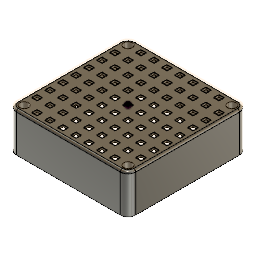
box (Autodesk Fusion 360 design; units mm, degrees)
Autodesk Fusion 360 part; units mm, degrees
sketch "Sketch1" plane through (0, 0, 0) normal (0, 0, 1) x (1, 0, 0) in component "Bottom"
  line L0 (50, 55) -> (-50, 55)
  line L1 (-55, 50) -> (-55, -50)
  line L2 (-50, -55) -> (50, -55)
  line L3 (55, -50) -> (55, 50)
  line L4 (55, 55) -> (-55, -55) construction
  line L5 (-55, 55) -> (55, -55) construction
  arc A0 (-50, 55) -> (-55, 50) centre (-50, 50) ccw
  arc A1 (55, 50) -> (50, 55) centre (50, 50) ccw
  arc A2 (50, -55) -> (55, -50) centre (50, -50) ccw
  arc A3 (-55, -50) -> (-50, -55) centre (-50, -50) ccw
  circle A4 centre (-50, 50) radius 2.25
  circle A5 centre (-50, 50) radius 5.85
  circle A6 centre (50, 50) radius 2.25
  circle A7 centre (50, 50) radius 5.85
  circle A8 centre (-50, -50) radius 2.25
  circle A9 centre (-50, -50) radius 5.85
  circle A10 centre (50, -50) radius 2.25
  circle A11 centre (50, -50) radius 5.85
  dimension "d1" = 110
  dimension "d2" = 110
  dimension "d3" = 5
  dimension "d33" = 4.5
  dimension "d34" = 3.6
  dimension "d37" = 100
  dimension "d38" = -100
  dimension "d39" = 5
  constraint perpendicular L0 L1
  constraint parallel L0 L2
  constraint parallel L1 L3
  constraint horizontal L0
  constraint coincident L4 origin
  constraint coincident L5 origin
  constraint coincident L5.start L1
  constraint coincident L5.start L0
  constraint tangent L1 A0
  constraint tangent L0 A0
  constraint coincident L4.start L0
  constraint coincident L4.start L3
  constraint tangent L0 A1
  constraint tangent L3 A1
  constraint equal A0 A1
  constraint coincident L5.end L3
  constraint coincident L5.end L2
  constraint tangent L3 A2
  constraint tangent L2 A2
  constraint equal A0 A2
  constraint coincident L4.end L2
  constraint coincident L4.end L1
  constraint tangent L2 A3
  constraint tangent L1 A3
  constraint equal A0 A3
  constraint coincident L5 A0.centre
  measures "d1" distance of L5.start L4.end
  measures "d2" distance of L4.end L5.end
  measures "d3" radius of A0
  measures "d33" diameter of A4
  measures "d39" distance of L1 A0.centre
extrude "Extrude1" add sketch "Sketch1" along normal blind 2 contours L0 L3 A1 A7 | L0 L1 L2 L3 A5 A7 A9 A11 | L0 L1 A0 A5 | L2 L3 A2 A11 | L1 L2 A3 A9 picked at (54.0091, 48.6623) picked at (-54.0091, 48.6623) picked at (54.0091, -48.6623) picked at (-54.0091, -48.6623) makes body 1 in component "Bottom"
sketch "Sketch2" plane through (0, 0, 2) normal (0, 0, 1) x (-1, 0, 0) in component "Bottom"
  arc A0 (55, 50) -> (50, 55) centre (50, 50) ccw
  line L0 (50, 55) -> (-50, 55)
  arc A1 (-50, 55) -> (-55, 50) centre (-50, 50) ccw
  line L1 (-55, 50) -> (-55, -50)
  arc A2 (-55, -50) -> (-50, -55) centre (-50, -50) ccw
  line L2 (-50, -55) -> (50, -55)
  arc A3 (50, -55) -> (55, -50) centre (50, -50) ccw
  line L3 (55, -50) -> (55, 50)
  line L4 (44, 50) -> (-44, 50)
  line L5 (-44, 50) -> (-44, 10.8)
  line L6 (-44, 10.8) -> (44, 10.8)
  line L7 (44, 10.8) -> (44, 50)
  line L8 (44, 50) -> (-44, 10.8) construction
  line L9 (-44, 50) -> (44, 10.8) construction
  line L10 (0, -55) -> (0, 55) construction
  line L11 (50, 55) -> (-50, 55)
  line L12 (-37.8, 44.5) -> (37.8, 44.5) construction
  line L13 (37.8, 44.5) -> (37.8, 16.3) construction
  line L14 (37.8, 16.3) -> (-37.8, 16.3) construction
  line L15 (-37.8, 16.3) -> (-37.8, 44.5) construction
  line L16 (-37.8, 44.5) -> (37.8, 16.3) construction
  line L17 (37.8, 44.5) -> (-37.8, 16.3) construction
  circle A4 centre (37.8, 16.3) radius 1.5
  circle A5 centre (-37.8, 44.5) radius 1.5
  line L18 (-41.5, 7) -> (41.5, 7)
  line L19 (41.5, 7) -> (41.5, -50)
  line L20 (41.5, -50) -> (-41.5, -50)
  line L21 (-41.5, -50) -> (-41.5, 7)
  line L22 (-41.5, 7) -> (41.5, -50) construction
  line L23 (41.5, 7) -> (-41.5, -50) construction
  line L24 (-50, -55) -> (50, -55)
  line L25 (45, 10.5) -> (45, -53.5) construction
  line L26 (45, -53.5) -> (-45, -53.5) construction
  line L27 (-45, -53.5) -> (-45, 10.5) construction
  line L28 (-45, 10.5) -> (45, 10.5) construction
  circle A6 centre (-45, -9) radius 1.5
  circle A7 centre (45, -34) radius 1.5
  line L29 (-45, -13.5) -> (-41.5, -13.5)
  line L30 (-45, -4.5) -> (-41.5, -4.5)
  arc A8 (-45, -4.5) -> (-45, -13.5) centre (-45, -9) ccw
  line L31 (45, -38.5) -> (41.5, -38.5)
  line L32 (45, -29.5) -> (41.5, -29.5)
  arc A9 (45, -38.5) -> (45, -29.5) centre (45, -34) ccw
  circle A10 centre (50, -50) radius 2.25
  circle A11 centre (-50, -50) radius 2.25
  circle A12 centre (50, 50) radius 2.25
  circle A13 centre (-50, 50) radius 2.25
  point P0 (0, 30.4)
  point P1 (0, 30.4)
  point P2 (0, -21.5)
  dimension "d6" = 88
  dimension "d7" = 39.2
  dimension "d9" = 5
  dimension "d10" = 28.2
  dimension "d11" = 75.6
  dimension "d12" = 3
  dimension "d13" = 3
  dimension "d19" = 57
  dimension "d20" = 83
  dimension "d21" = 5
  dimension "d22" = -3.5
  dimension "d23" = 3
  dimension "d24" = 16
  dimension "d25" = 3
  dimension "d26" = 16
  constraint perpendicular L4 L5
  constraint parallel L4 L6
  constraint parallel L5 L7
  constraint coincident L8 P1
  constraint coincident L9 P1
  constraint midpoint L2 L10.start
  constraint midpoint L0 L10.end
  constraint coincident P1 L10
  constraint vertical L5
  constraint perpendicular L12 L13
  constraint parallel L12 L14
  constraint parallel L13 L15
  constraint horizontal L12
  constraint coincident L16 P1
  constraint coincident L17 P1
  constraint coincident P1 P0
  constraint coincident L13.end L14.start
  constraint coincident L12.start L15.end
  constraint perpendicular L18 L19
  constraint parallel L18 L20
  constraint parallel L19 L21
  constraint horizontal L18
  constraint coincident L22 P2
  constraint coincident L23 P2
  constraint coincident L10 P2
  constraint coincident L27 A6.centre
  constraint coincident L25 A7.centre
  constraint coincident L27 L29.start
  constraint coincident L21 L29.end
  constraint tangent L29 A8
  constraint perpendicular L21 L29
  constraint coincident L27 L30.start
  constraint coincident L21 L30.end
  constraint tangent L30 A8
  constraint perpendicular L21 L30
  constraint concentric A6 A8
  constraint coincident L25 L31.start
  constraint coincident L19 L31.end
  constraint tangent L31 A9
  constraint perpendicular L19 L31
  constraint coincident L25 L32.start
  constraint coincident L19 L32.end
  constraint tangent L32 A9
  constraint perpendicular L19 L32
  constraint concentric A7 A9
  measures "d6" distance of L5.end L6.end
  measures "d7" distance of L4.end L5.end
  measures "d9" distance of L4 L11
  measures "d10" distance of L12.end L13.end
  measures "d11" distance of L13 L15
  measures "d12" diameter of A4
  measures "d13" diameter of A5
  measures "d19" distance of L18.end L19.end
  measures "d20" distance of L19.end L20.end
  measures "d21" distance of L20 L24
  measures "d23" diameter of A6
  measures "d24" vertical distance of L18.start A6.centre
  measures "d25" diameter of A7
  measures "d26" distance of L20 A7.centre
extrude "Extrude2" add sketch "Sketch2" along normal blind 1 contours L18 L19 L20 L21 | L21 L29 L30 A8 | L19 L31 L32 A9 bodies 1 in component "Bottom"
extrude "Extrude4" add sketch "Sketch2" along normal blind 3 contours L4 L5 L6 L7 bodies 1 in component "Bottom"
fillet "Fillet2" radius 4 4 edges at (44, -10.8, 3.5) (-44, -10.8, 3.5) (-44, -50, 3.5) (44, -50, 3.5) on bodies 1 in component "Bottom"
extrude "Extrude5" cut sketch "Sketch2" against normal through all contours A4 | A5 | A6 | A7 bodies 1 in component "Bottom"
ref_plane "WorkPlane1" through (0, 0, 36) normal (0, 0, 1) x (-1, 0, 0) in component "Cover"
sketch "Sketch1 (2)" plane through (0, 0, 36) normal (0, 0, 1) x (1, 0, 0) in component "Cover"
  circle A0 centre (37.8, -44.5) radius 1.5
  circle A1 centre (45, 9) radius 1.5
  circle A2 centre (-37.8, -16.3) radius 1.5
  circle A3 centre (-45, 34) radius 1.5
  circle A4 centre (-50, -50) radius 2.25
  circle A5 centre (-50, 50) radius 2.25
  circle A6 centre (50, -50) radius 2.25
  circle A7 centre (50, 50) radius 2.25
  arc A8 (-55, -50) -> (-50, -55) centre (-50, -50) ccw
  line L0 (-55, -50) -> (-55, 50)
  arc A9 (-50, 55) -> (-55, 50) centre (-50, 50) ccw
  line L1 (-50, 55) -> (50, 55)
  arc A10 (55, 50) -> (50, 55) centre (50, 50) ccw
  line L2 (55, 50) -> (55, -50)
  arc A11 (50, -55) -> (55, -50) centre (50, -50) ccw
  line L3 (50, -55) -> (-50, -55)
  arc A12 (-55.4, -50) -> (-50, -55.4) centre (-50, -50) ccw
  line L4 (50, -55.4) -> (-50, -55.4)
  arc A13 (50, -55.4) -> (55.4, -50) centre (50, -50) ccw
  line L5 (55.4, 50) -> (55.4, -50)
  arc A14 (55.4, 50) -> (50, 55.4) centre (50, 50) ccw
  line L6 (-50, 55.4) -> (50, 55.4)
  arc A15 (-50, 55.4) -> (-55.4, 50) centre (-50, 50) ccw
  line L7 (-55.4, -50) -> (-55.4, 50)
  arc A16 (-57.4, -50) -> (-50, -57.4) centre (-50, -50) ccw
  line L8 (50, -57.4) -> (-50, -57.4)
  arc A17 (50, -57.4) -> (57.4, -50) centre (50, -50) ccw
  line L9 (57.4, 50) -> (57.4, -50)
  arc A18 (57.4, 50) -> (50, 57.4) centre (50, 50) ccw
  line L10 (-50, 57.4) -> (50, 57.4)
  arc A19 (-50, 57.4) -> (-57.4, 50) centre (-50, 50) ccw
  line L11 (-57.4, -50) -> (-57.4, 50)
  dimension "d41" = -0.4
  dimension "d42" = -2.4
extrude "Extrude1'" add sketch "Sketch1 (2)" along normal blind 2 separate body contours A0 | A1 | A2 | A3 | A8 L0 A9 L1 A10 L2 A11 L3 | A12 L4 A13 L5 A14 L6 A15 L7 | A16 L8 A17 L9 A18 L10 A19 L11 makes body 2 in component "Cover"
sketch "Sketch2 (2)" plane through (0, 0, 36) normal (0, 0, 1) x (1, 0, 0) in component "Cover"
  circle A0 centre (-50, -50) radius 5.85
  circle A1 centre (50, -50) radius 5.85
  circle A2 centre (50, 50) radius 5.85
  circle A3 centre (-50, 50) radius 5.85
  circle A4 centre (50, -50) radius 2.25 construction
  circle A5 centre (-50, -50) radius 2.25 construction
  circle A6 centre (-50, 50) radius 2.25 construction
  circle A7 centre (50, 50) radius 2.25 construction
  line L0 (-57.4, 50) -> (-57.4, -50)
  line L1 (-57.4, -44.15) -> (-50, -44.15)
  line L2 (50, -57.4) -> (-50, -57.4)
  line L3 (-44.15, -50) -> (-44.15, -57.4)
  line L4 (44.15, -50) -> (44.15, -57.4)
  line L5 (57.4, -50) -> (57.4, 50)
  line L6 (50, -44.15) -> (57.4, -44.15)
  line L7 (50, 44.15) -> (57.4, 44.15)
  line L8 (-50, 57.4) -> (50, 57.4)
  line L9 (44.15, 50) -> (44.15, 57.4)
  line L10 (-50, 44.15) -> (-57.4, 44.15)
  line L11 (-44.15, 50) -> (-44.15, 57.4)
  circle A8 centre (-50, -50) radius 2.25
  circle A9 centre (-50, 50) radius 2.25
  circle A10 centre (50, 50) radius 2.25
  circle A11 centre (50, -50) radius 2.25
  arc A12 (50, -57.4) -> (57.4, -50) centre (50, -50) ccw
  line L12 (50, -57.4) -> (-50, -57.4)
  arc A13 (-57.4, -50) -> (-50, -57.4) centre (-50, -50) ccw
  line L13 (-57.4, -50) -> (-57.4, 50)
  arc A14 (-50, 57.4) -> (-57.4, 50) centre (-50, 50) ccw
  line L14 (-50, 57.4) -> (50, 57.4)
  arc A15 (57.4, 50) -> (50, 57.4) centre (50, 50) ccw
  line L15 (57.4, 50) -> (57.4, -50)
  constraint coincident L0 L1.start
  constraint coincident A0 L1.end
  constraint tangent A0 L1
  constraint perpendicular L0 L1
  constraint coincident A0 L3.start
  constraint coincident L2 L3.end
  constraint tangent A0 L3
  constraint perpendicular L2 L3
  constraint coincident A1 L4.start
  constraint coincident L2 L4.end
  constraint coincident A1 L6.start
  constraint coincident L5 L6.end
  constraint tangent A1 L6
  constraint perpendicular L5 L6
  constraint coincident A2 L7.start
  constraint coincident L5 L7.end
  constraint coincident A2 L9.start
  constraint coincident L8 L9.end
  constraint tangent A2 L9
  constraint perpendicular L8 L9
  constraint coincident A3 L10.start
  constraint coincident L0 L10.end
  constraint coincident A3 L11.start
  constraint coincident L8 L11.end
  constraint tangent A3 L10
  constraint tangent A3 L11
  constraint tangent A2 L7
  constraint tangent A1 L4
  constraint perpendicular L8 L11
  constraint perpendicular L0 L10
  constraint perpendicular L5 L7
  constraint perpendicular L2 L4
extrude "Extrude3" add sketch "Sketch2 (2)" against normal blind 34 contours A0 | A0 L0 L1 L2 L3 L12 A13 L13 | A1 L2 L4 L5 L6 A12 L12 L15 | A3 L0 L8 L10 L11 L13 A14 L14 | A1 | A3 | A2 L5 L7 L8 L9 L14 A15 L15 | A2 bodies 2 in component "Cover"
extrude "Extrude2'" add sketch "Sketch1 (2)" against normal up to surface (36 mm away) contours A16 L8 A17 L9 A18 L10 A19 L11 bodies 2 in component "Cover"
sketch "Sketch3" plane through (0, 0, 38) normal (0, 0, 1) x (-1, 0, 0) in component "Cover"
  circle A0 centre (-50, -50) radius 2.25
  circle A1 centre (-50, 50) radius 2.25
  circle A2 centre (50, -50) radius 2.25
  circle A3 centre (50, 50) radius 2.25
  arc A4 (-50, 57.4) -> (-57.4, 50) centre (-50, 50) ccw
  line L0 (-57.4, 50) -> (-57.4, -50)
  arc A5 (-57.4, -50) -> (-50, -57.4) centre (-50, -50) ccw
  line L1 (-50, -57.4) -> (50, -57.4)
  arc A6 (50, -57.4) -> (57.4, -50) centre (50, -50) ccw
  line L2 (57.4, -50) -> (57.4, 50)
  arc A7 (57.4, 50) -> (50, 57.4) centre (50, 50) ccw
  line L3 (50, 57.4) -> (-50, 57.4)
  circle A8 centre (50, -50) radius 4.1
  circle A9 centre (-50, -50) radius 4.1
  circle A10 centre (50, 50) radius 4.1
  circle A11 centre (-50, 50) radius 4.1
  dimension "d49" = 8.2
  dimension "d50" = 8.2
  dimension "d51" = 8.2
  dimension "d52" = 8.2
  constraint concentric A2 A8
  constraint concentric A0 A9
  constraint concentric A3 A10
  constraint concentric A1 A11
  measures "d49" diameter of A8
  measures "d50" diameter of A9
  measures "d51" diameter of A10
  measures "d52" diameter of A11
extrude "Extrude4'" cut sketch "Sketch3" against normal blind 30 contours A8 | A9 | A10 | A11 bodies 2 in component "Cover"
chamfer "Chamfer1" distance 1.8 angle 45 4 edges at (-52.0977, -50.8136, 8) (-52.0977, 49.1864, 8) (47.9023, 49.1864, 8) (47.9023, -50.8136, 8) on bodies 2 in component "Cover"
sketch "Sketch4" plane through (0, 0, 38) normal (0, 0, 1) x (-1, 0, 0) in component "Cover"
  circle A0 centre (50, -50) radius 4.1
  circle A1 centre (-50, -50) radius 4.1
  circle A2 centre (50, 50) radius 4.1
  circle A3 centre (-50, 50) radius 4.1
  arc A4 (-50, 57.4) -> (-57.4, 50) centre (-50, 50) ccw
  line L0 (-57.4, 50) -> (-57.4, -50)
  arc A5 (-57.4, -50) -> (-50, -57.4) centre (-50, -50) ccw
  line L1 (-50, -57.4) -> (50, -57.4)
  arc A6 (50, -57.4) -> (57.4, -50) centre (50, -50) ccw
  line L2 (57.4, -50) -> (57.4, 50)
  arc A7 (57.4, 50) -> (50, 57.4) centre (50, 50) ccw
  line L3 (50, 57.4) -> (-50, 57.4)
  line L4 (-2.5, -2.5) -> (2.5, -2.5)
  line L5 (2.5, -2.5) -> (2.5, 2.5)
  line L6 (2.5, 2.5) -> (-2.5, 2.5)
  line L7 (-2.5, 2.5) -> (-2.5, -2.5)
  line L8 (-2.5, -2.5) -> (2.5, 2.5) construction
  line L9 (2.5, -2.5) -> (-2.5, 2.5) construction
  line L10 (-35, -52.5) -> (-35, -47.5)
  line L11 (-40, -52.5) -> (-35, -52.5)
  line L12 (-40, -47.5) -> (-40, -52.5)
  line L13 (-35, -47.5) -> (-40, -47.5)
  line L14 (-22.5, -52.5) -> (-22.5, -47.5)
  line L15 (-27.5, -52.5) -> (-22.5, -52.5)
  line L16 (-27.5, -47.5) -> (-27.5, -52.5)
  line L17 (-22.5, -47.5) -> (-27.5, -47.5)
  line L18 (-10, -52.5) -> (-10, -47.5)
  line L19 (-15, -52.5) -> (-10, -52.5)
  line L20 (-15, -47.5) -> (-15, -52.5)
  line L21 (-10, -47.5) -> (-15, -47.5)
  line L22 (2.5, -52.5) -> (2.5, -47.5)
  line L23 (-2.5, -52.5) -> (2.5, -52.5)
  line L24 (-2.5, -47.5) -> (-2.5, -52.5)
  line L25 (2.5, -47.5) -> (-2.5, -47.5)
  line L26 (15, -52.5) -> (15, -47.5)
  line L27 (10, -52.5) -> (15, -52.5)
  line L28 (10, -47.5) -> (10, -52.5)
  line L29 (15, -47.5) -> (10, -47.5)
  line L30 (27.5, -52.5) -> (27.5, -47.5)
  line L31 (22.5, -52.5) -> (27.5, -52.5)
  line L32 (22.5, -47.5) -> (22.5, -52.5)
  line L33 (27.5, -47.5) -> (22.5, -47.5)
  line L34 (40, -52.5) -> (40, -47.5)
  line L35 (35, -52.5) -> (40, -52.5)
  line L36 (35, -47.5) -> (35, -52.5)
  line L37 (40, -47.5) -> (35, -47.5)
  line L38 (-47.5, -40) -> (-47.5, -35)
  line L39 (-52.5, -40) -> (-47.5, -40)
  line L40 (-52.5, -35) -> (-52.5, -40)
  line L41 (-47.5, -35) -> (-52.5, -35)
  line L42 (-35, -40) -> (-35, -35)
  line L43 (-40, -40) -> (-35, -40)
  line L44 (-40, -35) -> (-40, -40)
  line L45 (-35, -35) -> (-40, -35)
  line L46 (-22.5, -40) -> (-22.5, -35)
  line L47 (-27.5, -40) -> (-22.5, -40)
  line L48 (-27.5, -35) -> (-27.5, -40)
  line L49 (-22.5, -35) -> (-27.5, -35)
  line L50 (-10, -40) -> (-10, -35)
  line L51 (-15, -40) -> (-10, -40)
  line L52 (-15, -35) -> (-15, -40)
  line L53 (-10, -35) -> (-15, -35)
  line L54 (2.5, -40) -> (2.5, -35)
  line L55 (-2.5, -40) -> (2.5, -40)
  line L56 (-2.5, -35) -> (-2.5, -40)
  line L57 (2.5, -35) -> (-2.5, -35)
  line L58 (15, -40) -> (15, -35)
  line L59 (10, -40) -> (15, -40)
  line L60 (10, -35) -> (10, -40)
  line L61 (15, -35) -> (10, -35)
  line L62 (27.5, -40) -> (27.5, -35)
  line L63 (22.5, -40) -> (27.5, -40)
  line L64 (22.5, -35) -> (22.5, -40)
  line L65 (27.5, -35) -> (22.5, -35)
  line L66 (40, -40) -> (40, -35)
  line L67 (35, -40) -> (40, -40)
  line L68 (35, -35) -> (35, -40)
  line L69 (40, -35) -> (35, -35)
  line L70 (52.5, -40) -> (52.5, -35)
  line L71 (47.5, -40) -> (52.5, -40)
  line L72 (47.5, -35) -> (47.5, -40)
  line L73 (52.5, -35) -> (47.5, -35)
  line L74 (-47.5, -27.5) -> (-47.5, -22.5)
  line L75 (-52.5, -27.5) -> (-47.5, -27.5)
  line L76 (-52.5, -22.5) -> (-52.5, -27.5)
  line L77 (-47.5, -22.5) -> (-52.5, -22.5)
  line L78 (-35, -27.5) -> (-35, -22.5)
  line L79 (-40, -27.5) -> (-35, -27.5)
  line L80 (-40, -22.5) -> (-40, -27.5)
  line L81 (-35, -22.5) -> (-40, -22.5)
  line L82 (-22.5, -27.5) -> (-22.5, -22.5)
  line L83 (-27.5, -27.5) -> (-22.5, -27.5)
  line L84 (-27.5, -22.5) -> (-27.5, -27.5)
  line L85 (-22.5, -22.5) -> (-27.5, -22.5)
  line L86 (-10, -27.5) -> (-10, -22.5)
  line L87 (-15, -27.5) -> (-10, -27.5)
  line L88 (-15, -22.5) -> (-15, -27.5)
  line L89 (-10, -22.5) -> (-15, -22.5)
  line L90 (2.5, -27.5) -> (2.5, -22.5)
  line L91 (-2.5, -27.5) -> (2.5, -27.5)
  line L92 (-2.5, -22.5) -> (-2.5, -27.5)
  line L93 (2.5, -22.5) -> (-2.5, -22.5)
  line L94 (15, -27.5) -> (15, -22.5)
  line L95 (10, -27.5) -> (15, -27.5)
  line L96 (10, -22.5) -> (10, -27.5)
  line L97 (15, -22.5) -> (10, -22.5)
  line L98 (27.5, -27.5) -> (27.5, -22.5)
  line L99 (22.5, -27.5) -> (27.5, -27.5)
  line L100 (22.5, -22.5) -> (22.5, -27.5)
  line L101 (27.5, -22.5) -> (22.5, -22.5)
  line L102 (40, -27.5) -> (40, -22.5)
  line L103 (35, -27.5) -> (40, -27.5)
  line L104 (35, -22.5) -> (35, -27.5)
  line L105 (40, -22.5) -> (35, -22.5)
  line L106 (52.5, -27.5) -> (52.5, -22.5)
  line L107 (47.5, -27.5) -> (52.5, -27.5)
  line L108 (47.5, -22.5) -> (47.5, -27.5)
  line L109 (52.5, -22.5) -> (47.5, -22.5)
  line L110 (-47.5, -15) -> (-47.5, -10)
  line L111 (-52.5, -15) -> (-47.5, -15)
  line L112 (-52.5, -10) -> (-52.5, -15)
  line L113 (-47.5, -10) -> (-52.5, -10)
  line L114 (-35, -15) -> (-35, -10)
  line L115 (-40, -15) -> (-35, -15)
  line L116 (-40, -10) -> (-40, -15)
  line L117 (-35, -10) -> (-40, -10)
  line L118 (-22.5, -15) -> (-22.5, -10)
  line L119 (-27.5, -15) -> (-22.5, -15)
  line L120 (-27.5, -10) -> (-27.5, -15)
  line L121 (-22.5, -10) -> (-27.5, -10)
  line L122 (-10, -15) -> (-10, -10)
  line L123 (-15, -15) -> (-10, -15)
  line L124 (-15, -10) -> (-15, -15)
  line L125 (-10, -10) -> (-15, -10)
  line L126 (2.5, -15) -> (2.5, -10)
  line L127 (-2.5, -15) -> (2.5, -15)
  line L128 (-2.5, -10) -> (-2.5, -15)
  line L129 (2.5, -10) -> (-2.5, -10)
  line L130 (15, -15) -> (15, -10)
  line L131 (10, -15) -> (15, -15)
  line L132 (10, -10) -> (10, -15)
  line L133 (15, -10) -> (10, -10)
  line L134 (27.5, -15) -> (27.5, -10)
  line L135 (22.5, -15) -> (27.5, -15)
  line L136 (22.5, -10) -> (22.5, -15)
  line L137 (27.5, -10) -> (22.5, -10)
  line L138 (40, -15) -> (40, -10)
  line L139 (35, -15) -> (40, -15)
  line L140 (35, -10) -> (35, -15)
  line L141 (40, -10) -> (35, -10)
  line L142 (52.5, -15) -> (52.5, -10)
  line L143 (47.5, -15) -> (52.5, -15)
  line L144 (47.5, -10) -> (47.5, -15)
  line L145 (52.5, -10) -> (47.5, -10)
  line L146 (-47.5, -2.5) -> (-47.5, 2.5)
  line L147 (-52.5, -2.5) -> (-47.5, -2.5)
  line L148 (-52.5, 2.5) -> (-52.5, -2.5)
  line L149 (-47.5, 2.5) -> (-52.5, 2.5)
  line L150 (-35, -2.5) -> (-35, 2.5)
  line L151 (-40, -2.5) -> (-35, -2.5)
  line L152 (-40, 2.5) -> (-40, -2.5)
  line L153 (-35, 2.5) -> (-40, 2.5)
  line L154 (-22.5, -2.5) -> (-22.5, 2.5)
  line L155 (-27.5, -2.5) -> (-22.5, -2.5)
  line L156 (-27.5, 2.5) -> (-27.5, -2.5)
  line L157 (-22.5, 2.5) -> (-27.5, 2.5)
  line L158 (-10, -2.5) -> (-10, 2.5)
  line L159 (-15, -2.5) -> (-10, -2.5)
  line L160 (-15, 2.5) -> (-15, -2.5)
  line L161 (-10, 2.5) -> (-15, 2.5)
  line L162 (15, -2.5) -> (15, 2.5)
  line L163 (10, -2.5) -> (15, -2.5)
  line L164 (10, 2.5) -> (10, -2.5)
  line L165 (15, 2.5) -> (10, 2.5)
  line L166 (27.5, -2.5) -> (27.5, 2.5)
  line L167 (22.5, -2.5) -> (27.5, -2.5)
  line L168 (22.5, 2.5) -> (22.5, -2.5)
  line L169 (27.5, 2.5) -> (22.5, 2.5)
  line L170 (40, -2.5) -> (40, 2.5)
  line L171 (35, -2.5) -> (40, -2.5)
  line L172 (35, 2.5) -> (35, -2.5)
  line L173 (40, 2.5) -> (35, 2.5)
  line L174 (52.5, -2.5) -> (52.5, 2.5)
  line L175 (47.5, -2.5) -> (52.5, -2.5)
  line L176 (47.5, 2.5) -> (47.5, -2.5)
  line L177 (52.5, 2.5) -> (47.5, 2.5)
  line L178 (-47.5, 10) -> (-47.5, 15)
  line L179 (-52.5, 10) -> (-47.5, 10)
  line L180 (-52.5, 15) -> (-52.5, 10)
  line L181 (-47.5, 15) -> (-52.5, 15)
  line L182 (-35, 10) -> (-35, 15)
  line L183 (-40, 10) -> (-35, 10)
  line L184 (-40, 15) -> (-40, 10)
  line L185 (-35, 15) -> (-40, 15)
  line L186 (-22.5, 10) -> (-22.5, 15)
  line L187 (-27.5, 10) -> (-22.5, 10)
  line L188 (-27.5, 15) -> (-27.5, 10)
  line L189 (-22.5, 15) -> (-27.5, 15)
  line L190 (-10, 10) -> (-10, 15)
  line L191 (-15, 10) -> (-10, 10)
  line L192 (-15, 15) -> (-15, 10)
  line L193 (-10, 15) -> (-15, 15)
  line L194 (2.5, 10) -> (2.5, 15)
  line L195 (-2.5, 10) -> (2.5, 10)
  line L196 (-2.5, 15) -> (-2.5, 10)
  line L197 (2.5, 15) -> (-2.5, 15)
  line L198 (15, 10) -> (15, 15)
  line L199 (10, 10) -> (15, 10)
  line L200 (10, 15) -> (10, 10)
  line L201 (15, 15) -> (10, 15)
  line L202 (27.5, 10) -> (27.5, 15)
  line L203 (22.5, 10) -> (27.5, 10)
  line L204 (22.5, 15) -> (22.5, 10)
  line L205 (27.5, 15) -> (22.5, 15)
  line L206 (40, 10) -> (40, 15)
  line L207 (35, 10) -> (40, 10)
  line L208 (35, 15) -> (35, 10)
  line L209 (40, 15) -> (35, 15)
  line L210 (52.5, 10) -> (52.5, 15)
  line L211 (47.5, 10) -> (52.5, 10)
  line L212 (47.5, 15) -> (47.5, 10)
  line L213 (52.5, 15) -> (47.5, 15)
  line L214 (-47.5, 22.5) -> (-47.5, 27.5)
  line L215 (-52.5, 22.5) -> (-47.5, 22.5)
  line L216 (-52.5, 27.5) -> (-52.5, 22.5)
  line L217 (-47.5, 27.5) -> (-52.5, 27.5)
  line L218 (-35, 22.5) -> (-35, 27.5)
  line L219 (-40, 22.5) -> (-35, 22.5)
  line L220 (-40, 27.5) -> (-40, 22.5)
  line L221 (-35, 27.5) -> (-40, 27.5)
  line L222 (-22.5, 22.5) -> (-22.5, 27.5)
  line L223 (-27.5, 22.5) -> (-22.5, 22.5)
  line L224 (-27.5, 27.5) -> (-27.5, 22.5)
  line L225 (-22.5, 27.5) -> (-27.5, 27.5)
  line L226 (-10, 22.5) -> (-10, 27.5)
  line L227 (-15, 22.5) -> (-10, 22.5)
  line L228 (-15, 27.5) -> (-15, 22.5)
  line L229 (-10, 27.5) -> (-15, 27.5)
  line L230 (2.5, 22.5) -> (2.5, 27.5)
  line L231 (-2.5, 22.5) -> (2.5, 22.5)
  line L232 (-2.5, 27.5) -> (-2.5, 22.5)
  line L233 (2.5, 27.5) -> (-2.5, 27.5)
  line L234 (15, 22.5) -> (15, 27.5)
  line L235 (10, 22.5) -> (15, 22.5)
  line L236 (10, 27.5) -> (10, 22.5)
  line L237 (15, 27.5) -> (10, 27.5)
  line L238 (27.5, 22.5) -> (27.5, 27.5)
  line L239 (22.5, 22.5) -> (27.5, 22.5)
  line L240 (22.5, 27.5) -> (22.5, 22.5)
  line L241 (27.5, 27.5) -> (22.5, 27.5)
  line L242 (40, 22.5) -> (40, 27.5)
  line L243 (35, 22.5) -> (40, 22.5)
  line L244 (35, 27.5) -> (35, 22.5)
  line L245 (40, 27.5) -> (35, 27.5)
  line L246 (52.5, 22.5) -> (52.5, 27.5)
  line L247 (47.5, 22.5) -> (52.5, 22.5)
  line L248 (47.5, 27.5) -> (47.5, 22.5)
  line L249 (52.5, 27.5) -> (47.5, 27.5)
  line L250 (-47.5, 35) -> (-47.5, 40)
  line L251 (-52.5, 35) -> (-47.5, 35)
  line L252 (-52.5, 40) -> (-52.5, 35)
  line L253 (-47.5, 40) -> (-52.5, 40)
  line L254 (-35, 35) -> (-35, 40)
  line L255 (-40, 35) -> (-35, 35)
  line L256 (-40, 40) -> (-40, 35)
  line L257 (-35, 40) -> (-40, 40)
  line L258 (-22.5, 35) -> (-22.5, 40)
  line L259 (-27.5, 35) -> (-22.5, 35)
  line L260 (-27.5, 40) -> (-27.5, 35)
  line L261 (-22.5, 40) -> (-27.5, 40)
  line L262 (-10, 35) -> (-10, 40)
  line L263 (-15, 35) -> (-10, 35)
  line L264 (-15, 40) -> (-15, 35)
  line L265 (-10, 40) -> (-15, 40)
  line L266 (2.5, 35) -> (2.5, 40)
  line L267 (-2.5, 35) -> (2.5, 35)
  line L268 (-2.5, 40) -> (-2.5, 35)
  line L269 (2.5, 40) -> (-2.5, 40)
  line L270 (15, 35) -> (15, 40)
  line L271 (10, 35) -> (15, 35)
  line L272 (10, 40) -> (10, 35)
  line L273 (15, 40) -> (10, 40)
  line L274 (27.5, 35) -> (27.5, 40)
  line L275 (22.5, 35) -> (27.5, 35)
  line L276 (22.5, 40) -> (22.5, 35)
  line L277 (27.5, 40) -> (22.5, 40)
  line L278 (40, 35) -> (40, 40)
  line L279 (35, 35) -> (40, 35)
  line L280 (35, 40) -> (35, 35)
  line L281 (40, 40) -> (35, 40)
  line L282 (52.5, 35) -> (52.5, 40)
  line L283 (47.5, 35) -> (52.5, 35)
  line L284 (47.5, 40) -> (47.5, 35)
  line L285 (52.5, 40) -> (47.5, 40)
  line L286 (-35, 47.5) -> (-35, 52.5)
  line L287 (-40, 47.5) -> (-35, 47.5)
  line L288 (-40, 52.5) -> (-40, 47.5)
  line L289 (-35, 52.5) -> (-40, 52.5)
  line L290 (-22.5, 47.5) -> (-22.5, 52.5)
  line L291 (-27.5, 47.5) -> (-22.5, 47.5)
  line L292 (-27.5, 52.5) -> (-27.5, 47.5)
  line L293 (-22.5, 52.5) -> (-27.5, 52.5)
  line L294 (-10, 47.5) -> (-10, 52.5)
  line L295 (-15, 47.5) -> (-10, 47.5)
  line L296 (-15, 52.5) -> (-15, 47.5)
  line L297 (-10, 52.5) -> (-15, 52.5)
  line L298 (2.5, 47.5) -> (2.5, 52.5)
  line L299 (-2.5, 47.5) -> (2.5, 47.5)
  line L300 (-2.5, 52.5) -> (-2.5, 47.5)
  line L301 (2.5, 52.5) -> (-2.5, 52.5)
  line L302 (15, 47.5) -> (15, 52.5)
  line L303 (10, 47.5) -> (15, 47.5)
  line L304 (10, 52.5) -> (10, 47.5)
  line L305 (15, 52.5) -> (10, 52.5)
  line L306 (27.5, 47.5) -> (27.5, 52.5)
  line L307 (22.5, 47.5) -> (27.5, 47.5)
  line L308 (22.5, 52.5) -> (22.5, 47.5)
  line L309 (27.5, 52.5) -> (22.5, 52.5)
  line L310 (40, 47.5) -> (40, 52.5)
  line L311 (35, 47.5) -> (40, 47.5)
  line L312 (35, 52.5) -> (35, 47.5)
  line L313 (40, 52.5) -> (35, 52.5)
  dimension "d57" = 5
  dimension "d58" = 5
  dimension "d61" = 50
  dimension "d62" = 50
  constraint perpendicular L4 L5
  constraint parallel L4 L6
  constraint parallel L5 L7
  constraint horizontal L4
  constraint coincident L8 origin
  constraint coincident L9 origin
  measures "d57" distance of L5.end L6.end
  measures "d58" distance of L4.end L5.end
extrude "Extrude5'" cut sketch "Sketch4" against normal blind 2 contours L4 L5 L6 L7 | L10 L11 L12 L13 | L14 L15 L16 L17 | L18 L19 L20 L21 | L22 L23 L24 L25 | L26 L27 L28 L29 | L30 L31 L32 L33 | L34 L35 L36 L37 | L38 L39 L40 L41 | L42 L43 L44 L45 | L46 L47 L48 L49 | L50 L51 L52 L53 | L54 L55 L56 L57 | L58 L59 L60 L61 | L62 L63 L64 L65 | L66 L67 L68 L69 | L70 L71 L72 L73 | L74 L75 L76 L77 | L78 L79 L80 L81 | L82 L83 L84 L85 | L86 L87 L88 L89 | L90 L91 L92 L93 | L94 L95 L96 L97 | L98 L99 L100 L101 | L102 L103 L104 L105 | L106 L107 L108 L109 | L110 L111 L112 L113 | L114 L115 L116 L117 | L118 L119 L120 L121 | L122 L123 L124 L125 | L126 L127 L128 L129 | L130 L131 L132 L133 | L134 L135 L136 L137 | L138 L139 L140 L141 | L142 L143 L144 L145 | L146 L147 L148 L149 | L150 L151 L152 L153 | L154 L155 L156 L157 | L158 L159 L160 L161 | L162 L163 L164 L165 | L166 L167 L168 L169 | L170 L171 L172 L173 | L174 L175 L176 L177 | L178 L179 L180 L181 | L182 L183 L184 L185 | L186 L187 L188 L189 | L190 L191 L192 L193 | L194 L195 L196 L197 | L198 L199 L200 L201 | L202 L203 L204 L205 | L206 L207 L208 L209 | L210 L211 L212 L213 | L214 L215 L216 L217 | L218 L219 L220 L221 | L222 L223 L224 L225 | L226 L227 L228 L229 | L230 L231 L232 L233 | L234 L235 L236 L237 | L238 L239 L240 L241 | L242 L243 L244 L245 | L246 L247 L248 L249 | L250 L251 L252 L253 | L254 L255 L256 L257 | L258 L259 L260 L261 | L262 L263 L264 L265 | L266 L267 L268 L269 | L270 L271 L272 L273 | L274 L275 L276 L277 | L278 L279 L280 L281 | L282 L283 L284 L285 | L286 L287 L288 L289 | L290 L291 L292 L293 | L294 L295 L296 L297 | L298 L299 L300 L301 | L302 L303 L304 L305 | L306 L307 L308 L309 | L310 L311 L312 L313 bodies 2 in component "Cover"
sketch "Sketch5" plane through (-57.4, 0, 0) normal (-1, 0, 0) x (0, -1, 0) in component "Cover"
  line L0 (50, 0) -> (50, 38)
  line L1 (50, 38) -> (-50, 38)
  line L2 (-50, 38) -> (-50, 0)
  line L3 (-50, 0) -> (50, 0)
  line L4 (12.0023, 45.3404) -> (12.0023, -16.6596) construction
  line L5 (27.5, 4.5) -> (27.5, 0)
  line L6 (32.5, 4.5) -> (32.5, 0)
  line L7 (-50, 2) -> (50, 2)
  arc A0 (32.5, 4.5) -> (27.5, 4.5) centre (30, 4.5) ccw
  line L8 (-3.4953, 4.5) -> (-3.4953, 0)
  arc A1 (-3.4953, 4.5) -> (-8.4953, 4.5) centre (-5.9953, 4.5) ccw
  line L9 (-8.4953, 4.5) -> (-8.4953, 0)
  dimension "d65" = 5
  dimension "d66" = 2.5
  dimension "d67" = 20
  constraint vertical L4
  constraint coincident L3 L5.end
  constraint coincident L3 L6.end
  constraint tangent L5 A0
  constraint tangent L6 A0
  constraint perpendicular L5 L7
  constraint perpendicular L6 L7
  constraint symmetric L4 L5.start L8.start
  constraint symmetric L4 L5.end L8.end
  constraint symmetric L4 L6.start A1.end
  constraint symmetric L4 L6.end L9.end
  constraint symmetric L4 A0 A1
  measures "d65" diameter of A0
  measures "d66" distance of A0.centre L7
  measures "d67" distance of L0 A0.centre
extrude "Extrude6" cut sketch "Sketch5" against normal up to surface (2 mm away) contours L3 L5 L6 L7 | L5 L6 L7 A0 | L3 L7 L8 L9 | L7 L8 A1 L9 bodies 2 in component "Cover"
fillet "Fillet2'" radius 2 8 edges at (57.4, 0, 38) (55.2326, 55.2326, 38) (0, 57.4, 38) (-55.2326, 55.2326, 38) (-57.4, 0, 38) (-55.2326, -55.2326, 38) (0, -57.4, 38) (55.2326, -55.2326, 38) on bodies 2 in component "Cover"
fillet "Fillet4" radius 2 16 edges at (55.4, 0, 36) (0, -55.4, 36) (-55.4, 0, 36) (52.7, -44.15, 36) (45.8634, -45.8634, 36) (44.15, -52.7, 36) (0, 55.4, 36) (44.15, 52.7, 36) (45.8634, 45.8634, 36) (52.7, 44.15, 36) (-52.7, 44.15, 36) (-45.8634, 45.8634, 36) (-44.15, 52.7, 36) (-44.15, -52.7, 36) (-45.8634, -45.8634, 36) (-52.7, -44.15, 36) on bodies 2 in component "Cover"
component "Bottom" placed x (1, 0, 0) y (0, 1, 0) z (0, 0, 1) at (0, 0, 0)
component "Cover" placed x (1, 0, 0) y (0, 1, 0) z (0, 0, 1) at (0, 0, 0)
component "Component" placed x (1, 0, 0) y (0, 1, 0) z (0, 0, 1) at (0, 0, 0)
equation "d10 = d7 - ( ( 5.5 * 2 ) * 1 mm )"
equation "d11 = d6 - ( ( 6.2 * 2 ) * 1 mm )"
equation "d13 = d12"
equation "d25 = d23"
equation "d26 = d24"
equation "d39 = ( d1 - 100 mm ) / 2"
equation "d42 = d41 - 2 mm"
equation "d50 = d49"
equation "d51 = d49"
equation "d52 = d49"
